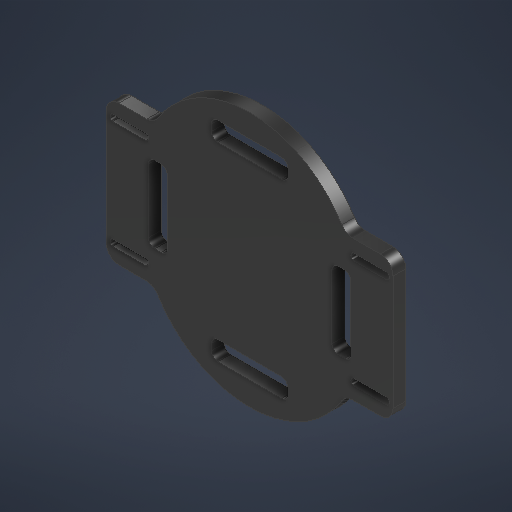
# Autodesk Inventor part: dudukansayapdrone
Saved by Autodesk Inventor 2026.1 (Build 301233000, 233)
## iProperties
Created: 2026-03-06
Part Number: dudukansayapdrone
Material: Generic
Document SubType Name: Modeling
Designer: ayjuni03
Density: 1 g/cm^3
Appearance: Default
Author: ayjuni03
Autodesk Inventor part; units mm, degrees
ref_plane "YZ Plane" through (0, 0, 0) normal (1, 0, 0) x (0, 1, 0)
ref_plane "XZ Plane" through (0, 0, 0) normal (0, 1, 0) x (-1, 0, 0)
ref_plane "XY Plane" through (0, 0, 0) normal (0, 0, 1) x (1, 0, 0)
sketch "Sketch1" plane through (0, 0, 0) normal (0, 0, 1) x (1, 0, 0)
  line L0 (0, 0) -> (-112.5, 0) construction
  line L1 (-112.5, 0) -> (112.5, 0) construction
  line L2 (0, 0) -> (0, 100) construction
  line L3 (0, 100) -> (0, -100) construction
  line L4 (0, 0) -> (-75, 0) construction
  line L5 (-75, 0) -> (-75, -55) construction
  line L6 (0, 0) -> (75, 0) construction
  line L7 (75, 0) -> (75, -55) construction
  arc A0 (-72.2813, -59.7687) -> (72.2813, -59.7687) centre (0, -15.4013) ccw
  line L8 (-112.5, 0) -> (-112.5, -45)
  line L9 (-102.5, -55) -> (-80.8039, -55)
  line L10 (80.8039, -55) -> (102.5, -55)
  line L11 (112.5, -45) -> (112.5, 0)
  line L12 (-75, 0) -> (-75, 55) construction
  line L13 (75, 0) -> (75, 55) construction
  arc A1 (72.2746, 59.7368) -> (-72.2746, 59.7368) centre (0, 15) ccw
  line L14 (-80.7775, 55) -> (-102.5, 55)
  line L15 (-112.5, 45) -> (-112.5, 0)
  line L16 (80.7775, 55) -> (102.5, 55)
  line L17 (112.5, 45) -> (112.5, 0)
  arc A2 (-102.5, 55) -> (-112.5, 45) centre (-102.5, 45) ccw
  arc A3 (-80.7775, 55) -> (-72.2746, 59.7368) centre (-80.7775, 65) ccw
  arc A4 (72.2746, 59.7368) -> (80.7775, 55) centre (80.7775, 65) ccw
  arc A5 (112.5, 45) -> (102.5, 55) centre (102.5, 45) ccw
  arc A6 (102.5, -55) -> (112.5, -45) centre (102.5, -45) ccw
  arc A7 (80.8039, -55) -> (72.2813, -59.7687) centre (80.8039, -65) ccw
  arc A8 (-72.2813, -59.7687) -> (-80.8039, -55) centre (-80.8039, -65) ccw
  arc A9 (-112.5, -45) -> (-102.5, -55) centre (-102.5, -45) ccw
  line L18 (-72.2746, 59.7368) -> (-61.9878, 53.5577) construction
  line L19 (-61.9878, 53.5577) -> (-58.8982, 58.7011)
  line L20 (-58.8982, 58.7011) -> (-33.1812, 43.2534)
  line L21 (-33.1812, 43.2534) -> (-36.2707, 38.11)
  line L22 (-36.2707, 38.11) -> (-61.9878, 53.5577)
  line L23 (-58.8982, 58.7011) -> (-56.8385, 62.1301)
  line L24 (-56.8385, 62.1301) -> (-31.1215, 46.6823)
  line L25 (-31.1215, 46.6823) -> (-28.0319, 51.8257)
  line L26 (-28.0319, 51.8257) -> (-53.749, 67.2735)
  line L27 (-53.749, 67.2735) -> (-56.8385, 62.1301)
  line L28 (75.9108, 56.2641) -> (66.1713, 49.254) construction
  line L29 (66.1713, 49.254) -> (62.6662, 54.1238) construction
  line L30 (62.6662, 54.1238) -> (38.3174, 36.5986) construction
  line L31 (38.3174, 36.5986) -> (41.8224, 31.7289) construction
  line L32 (41.8224, 31.7289) -> (66.1713, 49.254) construction
  line L33 (62.6662, 54.1238) -> (56.8245, 62.2401) construction
  line L34 (56.8245, 62.2401) -> (60.3296, 57.3703) construction
  line L35 (60.3296, 57.3703) -> (35.9829, 39.842) construction
  line L36 (35.9829, 39.842) -> (32.4779, 44.7118) construction
  line L37 (32.4779, 44.7118) -> (56.8245, 62.2401) construction
  line L38 (-75, -55) -> (-66.4238, -46.6067) construction
  line L39 (-66.4238, -46.6067) -> (-55.2326, -58.0416) construction
  line L40 (-55.2326, -58.0416) -> (-59.4293, -53.7535) construction
  line L41 (-59.4293, -53.7535) -> (-37.9887, -32.7702) construction
  line L42 (-37.9887, -32.7702) -> (-33.792, -37.0583) construction
  line L43 (-55.2326, -58.0416) -> (-33.792, -37.0583) construction
  line L44 (-66.4238, -46.6067) -> (-62.2271, -50.8948) construction
  line L45 (-62.2271, -50.8948) -> (-40.7865, -29.9114) construction
  line L46 (-40.7865, -29.9114) -> (-44.9832, -25.6233) construction
  line L47 (-44.9832, -25.6233) -> (-66.4238, -46.6067) construction
  line L48 (66.1713, -50.8948) -> (57.2172, -64.1547) construction
  line L49 (57.2172, -64.1547) -> (60.3546, -59.0403) construction
  line L50 (60.3546, -59.0403) -> (34.7828, -43.3533) construction
  line L51 (34.7828, -43.3533) -> (31.6454, -48.4676) construction
  line L52 (57.2172, -64.1547) -> (31.6454, -48.4676) construction
  line L53 (66.1713, -50.8948) -> (62.8135, -55.8672) construction
  line L54 (62.8135, -55.8672) -> (37.2417, -40.1802) construction
  line L55 (37.2417, -40.1802) -> (40.3791, -35.0658) construction
  line L56 (0, 100) -> (0, 82)
  line L57 (0, 82) -> (-25, 82)
  line L58 (-30, 82) -> (25, 82)
  line L59 (30, 77) -> (30, 72)
  line L60 (25, 67) -> (-25, 67)
  line L61 (-30, 72) -> (-30, 77)
  arc A10 (-25, 82) -> (-30, 77) centre (-25, 77) ccw
  arc A11 (-30, 72) -> (-25, 67) centre (-25, 72) ccw
  arc A12 (25, 67) -> (30, 72) centre (25, 72) ccw
  arc A13 (30, 77) -> (25, 82) centre (25, 77) ccw
  line L62 (0, -100) -> (0, -82) construction
  line L63 (0, -82) -> (-25, -82)
  line L64 (-30, -82) -> (25, -82)
  line L65 (30, -77) -> (30, -72)
  line L66 (25, -67) -> (-25, -67)
  line L67 (-30, -72) -> (-30, -77)
  arc A14 (-25, -67) -> (-30, -72) centre (-25, -72) ccw
  arc A15 (-30, -77) -> (-25, -82) centre (-25, -77) ccw
  arc A16 (25, -82) -> (30, -77) centre (25, -77) ccw
  arc A17 (30, -72) -> (25, -67) centre (25, -72) ccw
  line L68 (66.1713, -50.8948) -> (40.3791, -35.0658) construction
  line L69 (102.5, 55) -> (102.5, 45) construction
  line L70 (112.5, 45) -> (109.5, 45) construction
  line L71 (107.5, 45) -> (81.5, 45)
  line L72 (79.5, 43) -> (79.5, 42)
  line L73 (81.5, 40) -> (107.5, 40)
  line L74 (109.5, 42) -> (109.5, 43)
  arc A18 (81.5, 45) -> (79.5, 43) centre (81.5, 43) ccw
  arc A19 (79.5, 42) -> (81.5, 40) centre (81.5, 42) ccw
  arc A20 (107.5, 40) -> (109.5, 42) centre (107.5, 42) ccw
  arc A21 (109.5, 43) -> (107.5, 45) centre (107.5, 43) ccw
  line L75 (102.5, -45) -> (102.5, -55) construction
  line L76 (112.5, -45) -> (109.5, -45) construction
  line L77 (107.5, -45) -> (81.5, -45)
  line L78 (79.5, -43) -> (79.5, -42)
  line L79 (81.5, -40) -> (107.5, -40)
  line L80 (109.5, -42) -> (109.5, -43)
  arc A22 (79.5, -43) -> (81.5, -45) centre (81.5, -43) ccw
  arc A23 (81.5, -40) -> (79.5, -42) centre (81.5, -42) ccw
  arc A24 (107.5, -45) -> (109.5, -43) centre (107.5, -43) ccw
  arc A25 (109.5, -42) -> (107.5, -40) centre (107.5, -42) ccw
  line L81 (79.5, -40) -> (79.5, -30) construction
  line L82 (79.5, 40) -> (79.5, 30) construction
  line L83 (74.5, 30) -> (69.5, 30)
  line L84 (64.5, 25) -> (64.5, -25)
  line L85 (69.5, -30) -> (74.5, -30)
  line L86 (79.5, 25) -> (79.5, -25)
  arc A26 (69.5, 30) -> (64.5, 25) centre (69.5, 25) ccw
  arc A27 (64.5, -25) -> (69.5, -30) centre (69.5, -25) ccw
  arc A28 (74.5, -30) -> (79.5, -25) centre (74.5, -25) ccw
  arc A29 (79.5, 25) -> (74.5, 30) centre (74.5, 25) ccw
  line L87 (-102.5, -55) -> (-102.5, -45) construction
  line L88 (-112.5, -45) -> (-109.5, -45) construction
  line L89 (-107.5, -45) -> (-81.5, -45)
  line L90 (-79.5, -43) -> (-79.5, -42)
  line L91 (-81.5, -40) -> (-107.5, -40)
  line L92 (-109.5, -42) -> (-109.5, -43)
  arc A30 (-107.5, -40) -> (-109.5, -42) centre (-107.5, -42) ccw
  arc A31 (-109.5, -43) -> (-107.5, -45) centre (-107.5, -43) ccw
  arc A32 (-81.5, -45) -> (-79.5, -43) centre (-81.5, -43) ccw
  arc A33 (-79.5, -42) -> (-81.5, -40) centre (-81.5, -42) ccw
  line L93 (-102.5, 55) -> (-102.5, 45) construction
  line L94 (-112.5, 45) -> (-109.5, 45) construction
  line L95 (-107.5, 45) -> (-81.5, 45)
  line L96 (-79.5, 43) -> (-79.5, 42)
  line L97 (-81.5, 40) -> (-107.5, 40)
  line L98 (-109.5, 42) -> (-109.5, 43)
  arc A34 (-107.5, 45) -> (-109.5, 43) centre (-107.5, 43) ccw
  arc A35 (-109.5, 42) -> (-107.5, 40) centre (-107.5, 42) ccw
  arc A36 (-81.5, 40) -> (-79.5, 42) centre (-81.5, 42) ccw
  arc A37 (-79.5, 43) -> (-81.5, 45) centre (-81.5, 43) ccw
  line L99 (-79.5, 40) -> (-79.5, 30) construction
  line L100 (-79.5, 25) -> (-79.5, -25) construction
  line L101 (-79.5, -40) -> (-79.5, -30) construction
  line L102 (-74.5, -30) -> (-69.5, -30)
  line L103 (-64.5, -25) -> (-64.5, 25)
  line L104 (-69.5, 30) -> (-74.5, 30)
  line L105 (-79.5, 30) -> (-79.5, -30)
  arc A38 (-74.5, 30) -> (-79.5, 25) centre (-74.5, 25) ccw
  arc A39 (-64.5, 25) -> (-69.5, 30) centre (-69.5, 25) ccw
  arc A40 (-69.5, -30) -> (-64.5, -25) centre (-69.5, -25) ccw
  arc A41 (-79.5, -25) -> (-74.5, -30) centre (-74.5, -25) ccw
  point P0 (112.5, -55)
  point P1 (30, 82)
  point P2 (30, 67)
  point P3 (30, -82)
  point P4 (30, -67)
  point P5 (79.5, 45)
  point P6 (79.5, -45)
  point P7 (64.5, 30)
  point P8 (-79.5, -45)
  point P9 (-79.5, 45)
  point P10 (-64.5, -30)
  dimension "d0" = 112.5
  dimension "d1" = 225
  dimension "d2" = 100
  dimension "d3" = 200
  dimension "d4" = 75
  dimension "d5" = 55
  dimension "d6" = 75
  dimension "d7" = 55
  dimension "d8" = 55
  dimension "d9" = 10
  dimension "d10" = 12
  dimension "d11" = 6
  dimension "d12" = 30
  dimension "d13" = 4
  dimension "d14" = 6
  dimension "d15" = 12
  dimension "d16" = 6
  dimension "d17" = 30
  dimension "d18" = 10
  dimension "d19" = 6
  dimension "d20" = 30
  dimension "d21" = 6
  dimension "d22" = 12
  dimension "d23" = 16
  dimension "d24" = 6
  dimension "d25" = 30
  dimension "d26" = 6
  dimension "d27" = 16
  dimension "d28" = 6
  dimension "d29" = 30
  dimension "d30" = 6
  dimension "d31" = 30
  dimension "d32" = 6
  dimension "d33" = 18
  dimension "d34" = 30
  dimension "d35" = 60
  dimension "d36" = 15
  dimension "d37" = 5
  dimension "d38" = 18
  dimension "d39" = 30
  dimension "d40" = 60
  dimension "d41" = 15
  dimension "d42" = 5
  dimension "d43" = 3
  dimension "d44" = 30
  dimension "d45" = 5
  dimension "d46" = 2
  dimension "d47" = 2
  dimension "d48" = 30
  dimension "d49" = 5
  dimension "d50" = 2
  dimension "d51" = 10
  dimension "d52" = 10
  dimension "d53" = 15
  dimension "d54" = 5
  dimension "d55" = 3
  dimension "d56" = 30
  dimension "d57" = 2
  dimension "d58" = 3
  dimension "d59" = 30
  dimension "d60" = 5
  dimension "d61" = 2
  dimension "d62" = 10
  dimension "d63" = 70
  constraints: 212 end point, 90 point on circle, 80 tangent, 75 point on line, 56 perpendicular, 42 centre point, 30 equal radius, 10 vertical, 8 horizontal, 2 parallel, 1 collinear
  measures "d0" distance of L0.start L0.end
  measures "d1" distance of L0.end L1.end
  measures "d2" distance of L0.start L2.end
  measures "d3" distance of L2.end L3.end
  measures "d4" distance of L0.start L4.end
  measures "d5" distance of L4.end L5.end
  measures "d6" distance of L0.start L6.end
  measures "d7" distance of L4.end L12.end
  measures "d8" distance of L6.end L13.end
  measures "d9" radius of A2
  measures "d10" distance of L18.start L18.end
  measures "d11" distance of L18.end L19.end
  measures "d12" distance of L19.end L20.end
  measures "d13" distance of L19.end L23.end
  measures "d14" distance of L24.end L25.end
  measures "d15" distance of L28.start L28.end
  measures "d16" distance of L28.end L29.end
  measures "d17" distance of L29.end L30.end
  measures "d18" distance of L29.end L33.end
  measures "d19" distance of L33.end L34.end
  measures "d20" distance of L34.end L35.end
  measures "d21" distance of L35.end L36.end
  measures "d22" distance of L5.end L38.end
  measures "d23" distance of L38.end L39.end
  measures "d24" distance of L39.end L40.end
  measures "d25" distance of L40.end L41.end
  measures "d26" distance of L38.end L44.end
  measures "d27" distance of L48.start L48.end
  measures "d28" distance of L48.end L49.end
  measures "d29" distance of L49.end L50.end
  measures "d30" distance of L48.start L53.end
  measures "d31" distance of L53.end L54.end
  measures "d32" distance of L54.end L55.end
  measures "d33" distance of L2.end L56.end
  measures "d34" distance of L56.end L58.start
  measures "d35" distance of L58.start point (30, 82)
  measures "d36" distance of point (30, 82) point (30, 67)
  measures "d37" radius of A10
  measures "d38" distance of L3.end L62.end
  measures "d39" distance of L62.end L64.start
  measures "d40" distance of L64.start point (30, -82)
  measures "d41" distance of point (30, -82) point (30, -67)
  measures "d42" radius of A14
  measures "d43" distance of L17.start L70.end
  measures "d44" distance of L70.end point (79.5, 45)
  measures "d45" distance of point (79.5, 45) L82.start
  measures "d46" radius of A18
  measures "d47" radius of A21
  measures "d48" distance of L76.end point (79.5, -45)
  measures "d49" distance of point (79.5, -45) L81.start
  measures "d50" radius of A22
  measures "d51" distance of L81.start L81.end
  measures "d52" distance of L82.start L82.end
  measures "d53" distance of L82.end point (64.5, 30)
  measures "d54" radius of A26
  measures "d55" distance of L8.end L88.end
  measures "d56" distance of L88.end point (-79.5, -45)
  measures "d57" radius of A30
  measures "d58" distance of L15.start L94.end
  measures "d59" distance of L94.end point (-79.5, 45)
  measures "d60" distance of point (-79.5, 45) L99.start
  measures "d61" radius of A34
  measures "d62" distance of L99.start L99.end
  measures "d63" distance of L99.end L101.start
extrude "Extrusion1" add sketch "Sketch1" along normal blind 10 contours A8 L9 A9 L8 L15 A2 L14 A3 A1 A4 L16 A5 L17 L11 A6 L10 A7 A0 | L27 L26 L25 L24 | L19 L20 L21 L22
body "Solid1"
